Autodesk Inventor part; units mm, degrees
(part 2 of 2)
sketch "Sketch8" plane through (0, 13, 3.5) normal (0, 0, 1) x (1, 0, 0)
  arc A0 (230.5556, 129.6111) -> (230.5556, 138.5) centre (230.5556, 134.0556) ccw projected
  arc A1 (230.5556, 101.8333) -> (230.5556, 110.7222) centre (230.5556, 106.2778) ccw projected
  line L0 (230.5556, 134.0556) -> (230.5556, 106.2778) construction
  line L1 (230.5556, 120.1667) -> (223.5444, 120.1667) construction
  line L2 (230.5556, 124.6111) -> (223.5444, 124.6111)
  line L3 (223.5444, 115.7222) -> (230.5556, 115.7222)
  arc A2 (230.5556, 115.7222) -> (230.5556, 124.6111) centre (230.5556, 120.1667) ccw
  arc A3 (223.5444, 124.6111) -> (223.5444, 115.7222) centre (223.5444, 120.1667) ccw
  line L4 (219.1, 120.1667) -> (219.1, 126.405) construction
  arc A4 (209.6556, 115.7222) -> (209.6556, 124.6111) centre (209.6556, 120.1667) ccw projected
  line L5 (209.6556, 120.1667) -> (214.1, 120.1667) construction
  line L6 (214.1, 120.1667) -> (214.1, 126.405) construction
  line L7 (230.5556, 129.6111) -> (202.6444, 129.6111) projected
  line L8 (0, 157) -> (0, 0) projected
  line L9 (0, 157) -> (360, 157) projected
  line L10 (230.5556, 96.8333) -> (223.5444, 96.8333)
  line L11 (230.5556, 92.3889) -> (223.5444, 92.3889) construction
  arc A5 (230.5556, 87.9444) -> (230.5556, 96.8333) centre (230.5556, 92.3889) ccw
  line L12 (223.5444, 87.9444) -> (230.5556, 87.9444)
  arc A6 (223.5444, 96.8333) -> (223.5444, 87.9444) centre (223.5444, 92.3889) ccw
  line L13 (230.5556, 69.0556) -> (223.5444, 69.0556)
  line L14 (230.5556, 64.6111) -> (223.5444, 64.6111) construction
  arc A7 (230.5556, 60.1667) -> (230.5556, 69.0556) centre (230.5556, 64.6111) ccw
  line L15 (223.5444, 60.1667) -> (230.5556, 60.1667)
  arc A8 (223.5444, 69.0556) -> (223.5444, 60.1667) centre (223.5444, 64.6111) ccw
  line L16 (230.5556, 41.2778) -> (223.5444, 41.2778)
  line L17 (230.5556, 36.8333) -> (223.5444, 36.8333) construction
  arc A9 (230.5556, 32.3889) -> (230.5556, 41.2778) centre (230.5556, 36.8333) ccw
  line L18 (223.5444, 32.3889) -> (230.5556, 32.3889)
  arc A10 (223.5444, 41.2778) -> (223.5444, 32.3889) centre (223.5444, 36.8333) ccw
  line L19 (42.4556, 124.6111) -> (35.4444, 124.6111)
  line L20 (42.4556, 120.1667) -> (35.4444, 120.1667) construction
  arc A11 (42.4556, 115.7222) -> (42.4556, 124.6111) centre (42.4556, 120.1667) ccw
  line L21 (35.4444, 115.7222) -> (42.4556, 115.7222)
  arc A12 (35.4444, 124.6111) -> (35.4444, 115.7222) centre (35.4444, 120.1667) ccw
  line L22 (42.4556, 96.8333) -> (35.4444, 96.8333)
  line L23 (42.4556, 92.3889) -> (35.4444, 92.3889) construction
  arc A13 (42.4556, 87.9444) -> (42.4556, 96.8333) centre (42.4556, 92.3889) ccw
  line L24 (35.4444, 87.9444) -> (42.4556, 87.9444)
  arc A14 (35.4444, 96.8333) -> (35.4444, 87.9444) centre (35.4444, 92.3889) ccw
  line L25 (42.4556, 69.0556) -> (35.4444, 69.0556)
  line L26 (42.4556, 64.6111) -> (35.4444, 64.6111) construction
  arc A15 (42.4556, 60.1667) -> (42.4556, 69.0556) centre (42.4556, 64.6111) ccw
  line L27 (35.4444, 60.1667) -> (42.4556, 60.1667)
  arc A16 (35.4444, 69.0556) -> (35.4444, 60.1667) centre (35.4444, 64.6111) ccw
  line L28 (42.4556, 41.2778) -> (35.4444, 41.2778)
  line L29 (42.4556, 36.8333) -> (35.4444, 36.8333) construction
  arc A17 (42.4556, 32.3889) -> (42.4556, 41.2778) centre (42.4556, 36.8333) ccw
  line L30 (35.4444, 32.3889) -> (42.4556, 32.3889)
  arc A18 (35.4444, 41.2778) -> (35.4444, 32.3889) centre (35.4444, 36.8333) ccw
  arc A19 (35.4444, 138.5) -> (35.4444, 129.6111) centre (35.4444, 134.0556) ccw projected
  line L31 (35.4444, 134.0556) -> (35.4444, 120.1667) construction
  arc A20 (209.6556, 32.3889) -> (209.6556, 41.2778) centre (209.6556, 36.8333) ccw projected
  line L32 (209.6556, 36.8333) -> (223.5444, 36.8333) construction
  point P0 (0, -13)
  point P1 (227.05, 120.1667)
  point P2 (219.1, 92.3889)
  point P3 (227.05, 92.3889)
  point P4 (219.1, 64.6111)
  point P5 (227.05, 64.6111)
  point P6 (219.1, 36.8333)
  point P7 (227.05, 36.8333)
  point P8 (31, 120.1667)
  point P9 (38.95, 120.1667)
  point P10 (31, 92.3889)
  point P11 (38.95, 92.3889)
  point P12 (31, 64.6111)
  point P13 (38.95, 64.6111)
  point P14 (31, 36.8333)
  point P15 (38.95, 36.8333)
  dimension "d133" = 5
  dimension "d134" = 5
  dimension "d137" = 27.7778
  dimension "d140" = 188.1
  constraints: 76 end point, 34 point on circle, 16 centre point, 6 tangent, 5 vertical, 4 horizontal, 2 midpoint, 1 equal radius, 1 parallel, 91 other
  measures "d133" distance between parallel lines of L6 L4
  measures "d134" distance between parallel lines of L7 L2
  measures "d137" distance of L2.start L10.start
  measures "d140" distance of L2.start L19.start
extrude "Extrusion8" cut sketch "Sketch8" against normal blind 10
sketch "Sketch9" plane through (0, 13, -186.5) normal (0, 0, -1) x (-1, 0, 0)
  arc A0 (-138.0455, 17.9091) -> (-138.0455, 10) centre (-138.0455, 13.9545) ccw projected
  arc A1 (-138.0455, 43.7273) -> (-138.0455, 35.8182) centre (-138.0455, 39.7727) ccw projected
  line L0 (-138.0455, 13.9545) -> (-138.0455, 39.7727) construction
  line L1 (-138.0455, 26.8636) -> (-128.4545, 26.8636) construction
  line L2 (-146.9556, 27.3889) -> (-119.0444, 27.3889) projected
  line L3 (-138.0455, 22.9091) -> (-128.4545, 22.9091)
  line L4 (-128.4545, 30.8182) -> (-138.0455, 30.8182)
  arc A2 (-138.0455, 30.8182) -> (-138.0455, 22.9091) centre (-138.0455, 26.8636) ccw
  arc A3 (-128.4545, 22.9091) -> (-128.4545, 30.8182) centre (-128.4545, 26.8636) ccw
  line L5 (-124.5, 26.8636) -> (-124.5, 19.6592) construction
  arc A4 (-115.5455, 30.8182) -> (-115.5455, 22.9091) centre (-115.5455, 26.8636) ccw projected
  line L6 (-115.5455, 26.8636) -> (-119.5, 26.8636) construction
  line L7 (-119.5, 26.8636) -> (-119.5, 22.136) construction
  line L8 (-138.0455, 17.9091) -> (-105.9545, 17.9091) projected
  line L9 (0, 0) -> (-360, 0) projected
  line L10 (0, 0) -> (0, 157) projected
  line L11 (-15.9545, 30.8182) -> (-25.5455, 30.8182)
  arc A5 (-15.9545, 22.9091) -> (-15.9545, 30.8182) centre (-15.9545, 26.8636) ccw
  arc A6 (-25.5455, 30.8182) -> (-25.5455, 22.9091) centre (-25.5455, 26.8636) ccw
  line L12 (-25.5455, 22.9091) -> (-15.9545, 22.9091)
  line L13 (-25.5455, 26.8636) -> (-15.9545, 26.8636) construction
  line L14 (-128.4545, 56.6364) -> (-138.0455, 56.6364)
  arc A7 (-128.4545, 48.7273) -> (-128.4545, 56.6364) centre (-128.4545, 52.6818) ccw
  arc A8 (-138.0455, 56.6364) -> (-138.0455, 48.7273) centre (-138.0455, 52.6818) ccw
  line L15 (-138.0455, 48.7273) -> (-128.4545, 48.7273)
  line L16 (-138.0455, 52.6818) -> (-128.4545, 52.6818) construction
  line L17 (-15.9545, 56.6364) -> (-25.5455, 56.6364)
  arc A9 (-15.9545, 48.7273) -> (-15.9545, 56.6364) centre (-15.9545, 52.6818) ccw
  arc A10 (-25.5455, 56.6364) -> (-25.5455, 48.7273) centre (-25.5455, 52.6818) ccw
  line L18 (-25.5455, 48.7273) -> (-15.9545, 48.7273)
  line L19 (-25.5455, 52.6818) -> (-15.9545, 52.6818) construction
  line L20 (-128.4545, 82.4545) -> (-138.0455, 82.4545)
  arc A11 (-128.4545, 74.5455) -> (-128.4545, 82.4545) centre (-128.4545, 78.5) ccw
  arc A12 (-138.0455, 82.4545) -> (-138.0455, 74.5455) centre (-138.0455, 78.5) ccw
  line L21 (-138.0455, 74.5455) -> (-128.4545, 74.5455)
  line L22 (-138.0455, 78.5) -> (-128.4545, 78.5) construction
  line L23 (-15.9545, 82.4545) -> (-25.5455, 82.4545)
  arc A13 (-15.9545, 74.5455) -> (-15.9545, 82.4545) centre (-15.9545, 78.5) ccw
  arc A14 (-25.5455, 82.4545) -> (-25.5455, 74.5455) centre (-25.5455, 78.5) ccw
  line L24 (-25.5455, 74.5455) -> (-15.9545, 74.5455)
  line L25 (-25.5455, 78.5) -> (-15.9545, 78.5) construction
  line L26 (-128.4545, 108.2727) -> (-138.0455, 108.2727)
  arc A15 (-128.4545, 100.3636) -> (-128.4545, 108.2727) centre (-128.4545, 104.3182) ccw
  arc A16 (-138.0455, 108.2727) -> (-138.0455, 100.3636) centre (-138.0455, 104.3182) ccw
  line L27 (-138.0455, 100.3636) -> (-128.4545, 100.3636)
  line L28 (-138.0455, 104.3182) -> (-128.4545, 104.3182) construction
  line L29 (-15.9545, 108.2727) -> (-25.5455, 108.2727)
  arc A17 (-15.9545, 100.3636) -> (-15.9545, 108.2727) centre (-15.9545, 104.3182) ccw
  arc A18 (-25.5455, 108.2727) -> (-25.5455, 100.3636) centre (-25.5455, 104.3182) ccw
  line L30 (-25.5455, 100.3636) -> (-15.9545, 100.3636)
  line L31 (-25.5455, 104.3182) -> (-15.9545, 104.3182) construction
  line L32 (-128.4545, 134.0909) -> (-138.0455, 134.0909)
  arc A19 (-128.4545, 126.1818) -> (-128.4545, 134.0909) centre (-128.4545, 130.1364) ccw
  arc A20 (-138.0455, 134.0909) -> (-138.0455, 126.1818) centre (-138.0455, 130.1364) ccw
  line L33 (-138.0455, 126.1818) -> (-128.4545, 126.1818)
  line L34 (-138.0455, 130.1364) -> (-128.4545, 130.1364) construction
  line L35 (-15.9545, 134.0909) -> (-25.5455, 134.0909)
  arc A21 (-15.9545, 126.1818) -> (-15.9545, 134.0909) centre (-15.9545, 130.1364) ccw
  arc A22 (-25.5455, 134.0909) -> (-25.5455, 126.1818) centre (-25.5455, 130.1364) ccw
  line L36 (-25.5455, 126.1818) -> (-15.9545, 126.1818)
  line L37 (-25.5455, 130.1364) -> (-15.9545, 130.1364) construction
  arc A23 (-15.9545, 10) -> (-15.9545, 17.9091) centre (-15.9545, 13.9545) ccw projected
  line L38 (-15.9545, 13.9545) -> (-15.9545, 26.8636) construction
  arc A24 (-115.5455, 134.0909) -> (-115.5455, 126.1818) centre (-115.5455, 130.1364) ccw projected
  line L39 (-115.5455, 130.1364) -> (-128.4545, 130.1364) construction
  point P0 (0, -13)
  point P1 (-133.25, 26.8636)
  point P2 (-12, 26.8636)
  point P3 (-20.75, 26.8636)
  point P4 (-124.5, 52.6818)
  point P5 (-133.25, 52.6818)
  point P6 (-12, 52.6818)
  point P7 (-20.75, 52.6818)
  point P8 (-124.5, 78.5)
  point P9 (-133.25, 78.5)
  point P10 (-12, 78.5)
  point P11 (-20.75, 78.5)
  point P12 (-124.5, 104.3182)
  point P13 (-133.25, 104.3182)
  point P14 (-12, 104.3182)
  point P15 (-20.75, 104.3182)
  point P16 (-124.5, 130.1364)
  point P17 (-133.25, 130.1364)
  point P18 (-12, 130.1364)
  point P19 (-20.75, 130.1364)
  dimension "d149" = 5
  dimension "d150" = 5
  dimension "d153" = 112.5
  dimension "d156" = 25.8182
  constraints: 92 end point, 42 point on circle, 20 centre point, 5 tangent, 5 vertical, 3 horizontal, 2 midpoint, 2 parallel, 1 equal radius, 117 other
  measures "d149" distance between parallel lines of L3 L8
  measures "d150" distance between parallel lines of L5 L7
  measures "d153" distance of L4.start L11.start
  measures "d156" distance of L4.start L14.start
extrude "Extrusion9" cut sketch "Sketch9" against normal blind 10
equation "\"d27\" = d26"
equation "\"d54\" = d40"
equation "\"d57\" = d37"
equation "\"d113\" = d112"
equation "\"d132\" = d131"
equation "\"d74\" = d65"
equation "\"d78\" = d68"
equation "\"d81\" = d71"
equation "\"d110\" = d128"
equation "\"d130\" = d129"
equation "\"d103\" = d95"
equation "\"d106\" = d98"
equation "\"d148\" = d145"
equation "\"d116\" = d115"
equation "\"d125\" = d115"
equation "\"d133\" = d134"
equation "\"d150\" = d149"
equation "\"d65\" = 25"
body "Solid1"
